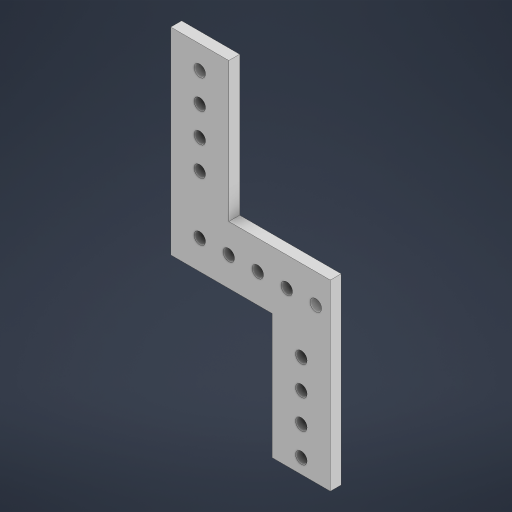
# Autodesk Inventor part: DVBS_007_Z-bracket1
Saved by Autodesk Inventor 2024 (Build 280153000, 153)
## iProperties
Created: 2024-07-29
Part Number: DVBS_007_Z-bracket1
Material: Generic
Document SubType Name: Modeling
Designer: sarav
Density: 1 g/cm^3
Appearance: Default
Author: sarav
Autodesk Inventor part; units mm, degrees
ref_plane "YZ Plane" through (0, 0, 0) normal (1, 0, 0) x (0, 1, 0)
ref_plane "XZ Plane" through (0, 0, 0) normal (0, 1, 0) x (-1, 0, 0)
ref_plane "XY Plane" through (0, 0, 0) normal (0, 0, 1) x (1, 0, 0)
sketch "Sketch1" plane through (0, 0, 0) normal (0, 0, 1) x (1, 0, 0)
  line L0 (-9.4525, -39.8078) -> (9.5975, -39.8078)
  line L1 (12.7725, -36.6328) -> (12.7725, 14.853)
  line L2 (-12.6275, 14.853) -> (-12.6275, -36.6328)
  line L3 (12.7725, 14.853) -> (12.7725, 40.253)
  line L4 (12.7725, 40.253) -> (-31.6775, 40.253)
  line L5 (-12.6275, 14.853) -> (-57.0775, 14.853)
  line L6 (-57.0775, 14.853) -> (-57.0775, 40.253)
  line L7 (-31.6775, 40.253) -> (-31.6775, 101.2638)
  line L8 (-31.6775, 101.2638) -> (-57.0775, 101.2638)
  line L9 (-57.0775, 101.2638) -> (-57.0775, 40.253)
  line L10 (-57.0775, 40.253) -> (-31.6775, 40.253)
  line L11 (-12.6275, -36.6328) -> (-12.6275, -39.8078)
  line L12 (-12.6275, -39.8078) -> (-9.4525, -39.8078)
  line L13 (9.5975, -39.8078) -> (12.7725, -39.8078)
  line L14 (12.7725, -39.8078) -> (12.7725, -36.6328)
  line L15 (-12.6275, 14.853) -> (12.7725, 14.853)
  dimension "d7" = 25.4
  dimension "d15" = 25.4
  dimension "d17" = 44.45
  dimension "d18" = 44.45
  dimension "d19" = 25.4
  dimension "d20" = 61.0108
  dimension "d21" = 25.4
  dimension "d23" = 54.6608
  constraints: 32 end point, 6 horizontal, 5 perpendicular, 4 vertical, 1 parallel, 1 point on line
  measures "d7" distance of L2.start L1.end
  measures "d15" distance of L1.end L3.end
  measures "d17" distance of L3.end L4.end
  measures "d18" distance of L2.start L5.end
  measures "d19" distance of L5.end L6.end
  measures "d20" distance of L4.end L7.end
  measures "d21" distance of L7.end L8.end
  measures "d23" distance of L13.end L1.end
extrude "Extrusion1" add sketch "Sketch1" along normal blind 4.7625
sketch "Sketch2" plane through (0, 0, 4.7625) normal (0, 0, 1) x (1, 0, 0)
  line L0 (-57.0775, 101.2638) -> (-57.0775, 14.853) projected
  line L1 (-57.0775, 14.853) -> (-12.6275, 14.853) projected
  line L2 (-12.6275, 14.853) -> (-12.6275, -39.8078) projected
  line L3 (-12.6275, -39.8078) -> (12.7725, -39.8078) projected
  line L4 (12.7725, -39.8078) -> (12.7725, 40.253) projected
  line L5 (12.7725, 40.253) -> (-31.6775, 40.253) projected
  line L6 (-31.6775, 40.253) -> (-31.6775, 101.2638) projected
  line L7 (-31.6775, 101.2638) -> (-57.0775, 101.2638) projected
  line L8 (-12.6275, 14.853) -> (12.7725, 14.853) construction
  circle A0 centre (0.0725, 4.6549) radius 2.5019
  line L9 (0.0725, 14.853) -> (0.0725, 7.1568) construction
  circle A1 centre (0.0725, -20.7451) radius 2.5019
  circle A2 centre (0.0725, -8.0451) radius 2.5019
  line L10 (0.0725, 2.153) -> (0.0725, -5.5432) construction
  line L11 (0.0725, -10.547) -> (0.0725, -18.2432) construction
  circle A3 centre (0.0725, -33.4451) radius 2.5019
  line L12 (0.0725, -23.247) -> (0.0725, -30.9432) construction
  line L13 (-57.0775, 101.2638) -> (-57.0775, 14.853) projected
  line L14 (12.7725, 14.853) -> (-57.0775, 14.853) construction
  line L15 (-57.0775, 14.853) -> (-57.0775, 40.253)
  line L16 (-57.0775, 40.253) -> (12.7725, 40.253) construction
  line L17 (12.7725, 40.253) -> (12.7725, 14.853)
  line L18 (-57.0775, 27.553) -> (12.7725, 27.553) construction
  circle A4 centre (6.4098, 27.553) radius 2.5019
  line L19 (8.9117, 27.553) -> (12.7725, 27.553)
  circle A5 centre (-6.2902, 27.553) radius 2.5019
  line L20 (-69.7775, 27.553) -> (0.0725, 27.553) construction
  circle A6 centre (-18.9902, 27.553) radius 2.5019
  line L21 (-82.4775, 27.553) -> (-12.6275, 27.553) construction
  circle A7 centre (-31.6902, 27.553) radius 2.5019
  line L22 (-95.1775, 27.553) -> (-25.3275, 27.553) construction
  circle A8 centre (-44.3902, 27.553) radius 2.5019
  line L23 (-107.8775, 27.553) -> (-38.0275, 27.553) construction
  line L24 (-44.3902, 40.253) -> (-44.3775, 101.2638) construction
  circle A9 centre (-44.3876, 52.9657) radius 2.5019
  line L25 (-44.3881, 50.4638) -> (-44.3902, 40.253)
  circle A10 centre (-44.3849, 65.6657) radius 2.5019
  circle A11 centre (-44.3823, 78.3657) radius 2.5019
  circle A12 centre (-44.3796, 91.0657) radius 2.5019
  point P0 (0, 0)
  point P1 (-3.7883, 27.553)
  point P2 (-16.4883, 27.553)
  point P3 (-29.1883, 27.553)
  point P4 (-41.8883, 27.553)
  point P5 (-44.3854, 63.1638)
  point P6 (-44.3828, 75.8638)
  point P7 (-44.3801, 88.5638)
  dimension "d34" = 5.0038
  dimension "d38" = 5.0038
  dimension "d47" = 5.0038
  dimension "d26" = 5.0038
  dimension "d29" = 7.6962
  dimension "d30" = 5.0038
  dimension "d31" = 5.0038
  dimension "d32" = 7.6962
  dimension "d33" = 7.6962
  dimension "d35" = 7.6962
  dimension "d37" = 25.4
  dimension "d39" = 3.8608
  dimension "d42" = 12.7
  dimension "d48" = 10.2108
  dimension "d51" = 12.7
  constraints: 34 end point, 23 point on line, 6 horizontal, 6 point on circle, 5 horizontal alignment, 4 midpoint, 3 centre point, 3 collinear, 3 parallel, 3 vertical, 2 perpendicular, 1 vertical alignment, 54 other
  measures "d26" diameter of A0
  measures "d29" distance of L9.start L9.end
  measures "d30" diameter of A1
  measures "d31" diameter of A2
  measures "d32" distance of L10.start L10.end
  measures "d33" distance of L11.start L11.end
  measures "d35" distance of L12.start L12.end
  measures "d37" distance of L8.end L4.end
  measures "d39" distance of L19.start L18.end
  measures "d42" distance of point (6.41, 27.553) point (-6.29, 27.553)
  measures "d48" distance of L25.start L24.start
  measures "d51" distance of point (-44.388, 52.966) point (-44.385, 65.666)
extrude "Extrusion2" cut sketch "Sketch2" against normal through all contours A0 | A1 | A2 | A3 | A4 | A5 | A6 | A7 | A8 | A9 | A10 | A11 | A12
body "Solid1"
